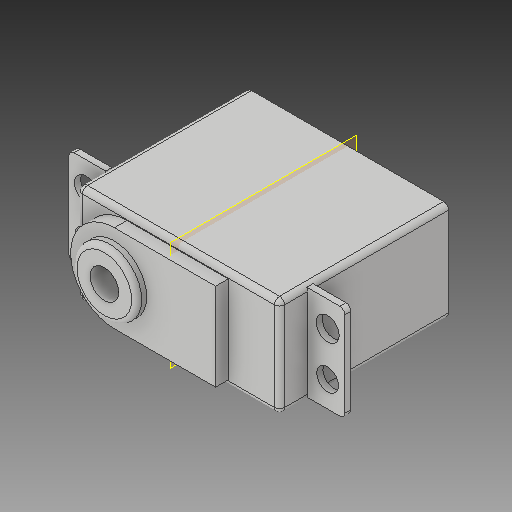
# Autodesk Inventor part: Corps
Saved by Autodesk Inventor 2018 (Build 220112000, 112)
## iProperties
Created: 2017-10-08
Part Number: Corps
Material: Generic
Document SubType Name: Modeling
Designer: liamg
Density: 1 g/cm^3
Appearance: Default
Mass: 28.3577 g
Surface Area: 65.1406 cm^2
Volume: 28.3577 cm^3
Author: liamg
Autodesk Inventor part; units mm, degrees
ref_plane "YZ Plane" through (0, 0, 0) normal (1, 0, 0) x (0, 1, 0)
ref_plane "XZ Plane" through (0, 0, 0) normal (0, 1, 0) x (-1, 0, 0)
ref_plane "XY Plane" through (0, 0, 0) normal (0, 0, 1) x (1, 0, 0)
sketch "Sketch1" plane through (0, 0, 0) normal (0, 0, 1) x (1, 0, 0)
  line L0 (-20.125, 9.85) -> (20.125, 9.85)
  line L1 (20.125, 9.85) -> (20.125, -9.85)
  line L2 (20.125, -9.85) -> (-20.125, -9.85)
  line L3 (-20.125, -9.85) -> (-20.125, 9.85)
  line L4 (-20.125, 9.85) -> (20.125, -9.85) construction
  line L5 (20.125, 9.85) -> (-20.125, -9.85) construction
  point P0 (0, 0)
  dimension "d0" = 40.25
  dimension "d1" = 19.7
  constraints: 12 end point, 2 midpoint, 2 parallel, 1 horizontal, 1 perpendicular
  measures "d0" distance of L1.end L2.end
  measures "d1" distance of L0.end L1.end
extrude "Extrusion1" add sketch "Sketch1" along normal blind 33.7
sketch "Sketch5" plane through (20.125, -9.85, 0) normal (1, 0, 0) x (0, 0, -1)
  line L0 (-33.7, 0) -> (-33.7, 19.7) construction
  line L1 (0, 0) -> (-33.7, 0) construction
  line L2 (0, 19.7) -> (-33.7, 19.7) construction
  line L3 (0, 19.7) -> (0, 0) construction
  line L4 (-33.7, 19.7) -> (-33.7, 0) construction
  line L5 (-33.7, 9.85) -> (0, 9.85) construction
  line L6 (0, 0) -> (0, 19.7) projected
  line L7 (-26.8226, 9.85) -> (-26.8226, 0.375) construction
  line L8 (-26.8226, 9.85) -> (-26.8226, 19.325) construction
  line L9 (-26.8226, 9.85) -> (-28.0526, 9.85) construction
  line L10 (-28.0526, 0.375) -> (-26.8226, 0.375)
  line L11 (-26.8226, 0.375) -> (-26.8226, 19.325)
  line L12 (-26.8226, 19.325) -> (-28.0526, 19.325)
  line L13 (-28.0526, 19.325) -> (-28.0526, 0.375)
  line L14 (-28.0526, 0.375) -> (-26.8226, 19.325) construction
  line L15 (-26.8226, 0.375) -> (-28.0526, 19.325) construction
  point P0 (-27.4376, 9.85)
  dimension "d11" = 1.23
  constraints: 20 end point, 4 midpoint, 4 perpendicular, 2 parallel, 2 point on line, 1 horizontal, 1 vertical
  measures "d11" distance of L7.start L9.end
extrude "Extrusion2" add sketch "Sketch5" along normal blind 7.36
fillet "Fillet1" radius 1 1 edges at (27.485, 9.475, 27.4376)
fillet "Fillet2" radius 1 1 edges at (27.485, -9.475, 27.4376)
fillet "Fillet3" radius 1 8 edges at (20.125, 9.85, 16.85) (20.125, -9.85, 16.85) (-20.125, 9.85, 16.85) (-20.125, -9.85, 16.85) (-20.125, 0, 33.7) (0, -9.85, 33.7) (20.125, 0, 33.7) (0, 9.85, 33.7)
ref_plane "Work Plane1" through (0, -8.85, 0) normal (1, 0, 0) x (0, 0, -1)
sketch "Sketch6" plane through (27.485, -8.475, 28.0526) normal (0, 0, 1) x (1, 0, 0)
  line L0 (0, 16.95) -> (0, 0) construction
  arc A0 (-1, -1) -> (0, 0) centre (-1, 0) ccw construction
  line L1 (-7.5794, -1) -> (-1, -1) construction
  line L2 (-1, 17.95) -> (-7.5794, 17.95) construction
  arc A1 (0, 16.95) -> (-1, 17.95) centre (-1, 16.95) ccw construction
  line L3 (0, 8.475) -> (-6.8446, 8.475) construction
  line L4 (-3.42, -1) -> (-3.42, 17.95) construction
  line L5 (0, 4.115) -> (-6.8446, 4.115) construction
  line L6 (0, 12.835) -> (-6.8446, 12.835) construction
  circle A2 centre (-3.4223, 4.115) radius 2.18
  circle A3 centre (-3.4223, 12.835) radius 2.3
  point P0 (-27.485, 8.475)
  dimension "d17" = 3.42
  dimension "d18" = 4.36
  dimension "d19" = 4.36
  dimension "d20" = 4.36
  dimension "d21" = 4.6
  constraints: 8 end point, 4 point on line, 3 midpoint, 3 perpendicular, 2 centre point, 1 horizontal
  measures "d17" distance between parallel lines of L0 L4
  measures "d18" distance between parallel lines of L3 L5
  measures "d19" distance between parallel lines of L3 L6
  measures "d20" diameter of A2
  measures "d21" diameter of A3
extrude "Extrusion3" cut sketch "Sketch6" against normal up to next
mirror "Mirror1" about plane through (0, -8.85, 0) normal (1, 0, 0) of "Extrusion2", "Extrusion3"
fillet "Fillet4" radius 1 2 edges at (-27.485, 9.475, 27.4376) (-27.485, -9.475, 27.4376)
sketch "Sketch7" plane through (-20.125, -8.85, 0) normal (-1, 0, 0) x (0, 0, 1)
  line L0 (26.8226, 0.375) -> (26.8226, 17.325) construction
  line L1 (0, 17.7) -> (26.8226, 17.7) construction
  line L2 (26.8226, 0) -> (0, 0) construction
  line L3 (0, 0) -> (0, 17.7) construction
  line L4 (7.54, 15.6992) -> (7.54, 1.4892) construction
  line L5 (7.54, 8.5942) -> (9.39, 8.5942) construction
  line L6 (11.24, 11.8242) -> (7.54, 11.8242)
  line L7 (7.54, 11.8242) -> (7.54, 5.3642)
  line L8 (7.54, 5.3642) -> (11.24, 5.3642)
  line L9 (11.24, 5.3642) -> (11.24, 11.8242)
  line L10 (11.24, 11.8242) -> (7.54, 5.3642) construction
  line L11 (7.54, 11.8242) -> (11.24, 5.3642) construction
  point P0 (0, 8.85)
  dimension "d25" = 7.54
  dimension "d26" = 1.85
  dimension "d27" = 6.46
  constraints: 16 end point, 3 midpoint, 2 horizontal, 2 parallel, 1 perpendicular, 1 point on line, 1 vertical
  measures "d25" distance between parallel lines of L3 L4
  measures "d26" distance of L5.start L5.end
  measures "d27" distance of L7.end L6.end
extrude "Extrusion4" add sketch "Sketch7" along normal blind 5.6
fillet "Fillet5" radius 1 8 edges at (-25.725, -0.2558, 11.24) (-22.925, -3.4858, 11.24) (-22.925, -3.4858, 7.54) (-25.725, -3.4858, 9.39) (-25.725, 2.9742, 9.39) (-25.725, -0.2558, 7.54) (-22.925, 2.9742, 11.24) (-22.925, 2.9742, 7.54)
sketch "Sketch8" plane through (0, 0, 33.7) normal (0, 0, 1) x (1, 0, 0)
  line L0 (-19.125, -8.85) -> (-19.125, 8.85) construction
  line L1 (19.125, -8.85) -> (-19.125, -8.85) construction
  line L2 (-19.125, 8.85) -> (19.125, 8.85) construction
  circle A0 centre (-10.275, 0) radius 8.85 construction
  arc A1 (-10.275, 8.7102) -> (-10.275, -8.7102) centre (-10.275, 0) ccw
  line L3 (-10.275, -8.7102) -> (9.8883, -8.7102)
  line L4 (9.8883, -8.7102) -> (9.8883, 7.9063)
  line L5 (-10.275, 8.7102) -> (9.8883, 8.7102)
  line L6 (9.8883, 8.7102) -> (9.8883, 7.8736)
  point P0 (0, 0)
  constraints: 8 end point, 2 centre point, 2 point on circle, 1 coincident, 1 horizontal, 1 parallel, 1 perpendicular, 1 point on line, 1 tangent
extrude "Extrusion5" add sketch "Sketch8" along normal blind 2.5
sketch "Sketch9" plane through (0, 0, 36.2) normal (0, 0, 1) x (1, 0, 0)
  arc A0 (-10.275, 8.7102) -> (-10.275, -8.7102) centre (-10.275, 0) ccw construction
  circle A1 centre (-10.275, 0) radius 6.44
  point P0 (0, 0)
  dimension "d34" = 12.88
  constraints: 1 centre point, 1 coincident
  measures "d34" diameter of A1
extrude "Extrusion6" add sketch "Sketch9" along normal blind 2
fillet "Fillet6" radius 1 1 edges at (-16.715, 0, 38.2)
sketch "Sketch10" plane through (-10.275, 0, 38.2) normal (0, 0, 1) x (1, 0, 0)
  circle A0 centre (0, 0) radius 2.855
  point P0 (10.275, 0)
  dimension "d38" = 5.71
  constraints: 1 centre point
  measures "d38" diameter of A0
extrude "Extrusion7" cut sketch "Sketch10" against normal blind 5
body "Solid1"
